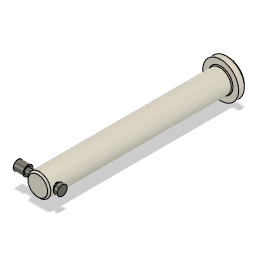
0.885.2200 - Axe pied de hauban - IGTE 21482_225065 (Autodesk Fusion 360 design; units mm, degrees)
Autodesk Fusion 360 part; units mm, degrees
sketch "Sketch1" plane through (0, 0, 0) normal (0, 0, 1) x (1, 0, 0)
  circle A0 centre (0, 0) radius 11
  dimension "d1" = 22
  constraint coincident A0.centre origin
  measures "d1" diameter of A0
extrude "Extrude1" add sketch "Sketch1" along normal blind 4.5 makes body 1
chamfer "Chamfer1" distance 1 angle 45 1 edges at (-10.2556, -3.9778, 0) on bodies 1
sketch "Sketch2" plane through (0, 0, 4.5) normal (0, 0, 1) x (1, 0, 0)
  circle A0 centre (0, 0) radius 11
  circle A1 centre (0, 0) radius 7
  dimension "d5" = 14
  constraint coincident A0.centre A1.centre
  measures "d5" diameter of A1
extrude "Extrude2" add sketch "Sketch2" along normal blind 112 contours A1 bodies 1
fillet "Fillet1" radius 0.5 1 edges at (-6.5263, 2.5313, 4.5) on bodies 1
sketch "Sketch3" plane through (0, 0, 0) normal (1, 0, 0) x (0, 0, -1)
  line L0 (-116.5, 0) -> (-111.5, 0) construction
  circle A0 centre (-111.5, 0) radius 2.5
  point P0 (-116.5, 0)
  dimension "d9" = 5
  dimension "d10" = 5
  constraint coincident P0 L0.start
  constraint coincident L0.end A0.centre
  measures "d9" distance of P0 L0.end
  measures "d10" diameter of A0
extrude "Extrude3" cut sketch "Sketch3" along normal through all and the other way through all bodies 1
chamfer "Chamfer2" distance 1 angle 45 1 edges at (-6.5263, -2.5313, 116.5) on bodies 1
sketch "Sketch4" plane through (0, 0, 0) normal (1, 0, 0) x (0, 0, -1)
  spline S0 degree 3 poles (-111.5, 2.5) (-111.1829, 2.5) (-110.8469, 2.4361) (-110.2319, 2.1801) (-109.9527, 1.9882) (-109.5119, 1.5474) (-109.3199, 1.2682) (-109.0639, 0.653) (-109, 0.3169) (-109, -0.3169) (-109.0639, -0.653) (-109.3199, -1.2682) (-109.5119, -1.5474) (-109.9527, -1.9882) (-110.2319, -2.1801) (-110.8469, -2.4361) (-111.1829, -2.5) (-111.8171, -2.5) (-112.1531, -2.4361) (-112.7681, -2.1801) (-113.0473, -1.9882) (-113.4881, -1.5474) (-113.6801, -1.2682) (-113.9361, -0.653) (-114, -0.3169) (-114, 0.3169) (-113.9361, 0.653) (-113.6801, 1.2682) (-113.4881, 1.5474) (-113.0473, 1.9882) (-112.7681, 2.1801) (-112.1531, 2.4361) (-111.8171, 2.5) (-111.5, 2.5) knots 0 0 0 0 0.095117 0.095117 0.190234 0.190234 0.285292 0.285292 0.38035 0.38035 0.475408 0.475408 0.570466 0.570466 0.665583 0.665583 0.7607 0.7607 0.855818 0.855818 0.950935 0.950935 1.045993 1.045993 1.141051 1.141051 1.236109 1.236109 1.331167 1.331167 1.426284 1.426284 1.521401 1.521401 1.521401 1.521401
  spline S1 degree 3 poles (-111.5, 2.2) (-111.2233, 2.2) (-110.9233, 2.1429) (-110.6547, 2.0311) (-110.3859, 1.9193) (-110.1368, 1.7481) (-109.9444, 1.5556) (-109.752, 1.3633) (-109.5808, 1.1141) (-109.4689, 0.8453) (-109.357, 0.5766) (-109.3, 0.2765) (-109.3, 0) (-109.3, -0.2765) (-109.357, -0.5766) (-109.4689, -0.8453) (-109.5808, -1.1141) (-109.752, -1.3633) (-109.9444, -1.5556) (-110.1368, -1.7481) (-110.3859, -1.9193) (-110.6547, -2.0311) (-110.9233, -2.1429) (-111.2233, -2.2) (-111.5, -2.2) (-111.7767, -2.2) (-112.0767, -2.1429) (-112.3453, -2.0311) (-112.6141, -1.9193) (-112.8632, -1.7481) (-113.0556, -1.5556) (-113.248, -1.3633) (-113.4192, -1.1141) (-113.5311, -0.8453) (-113.643, -0.5766) (-113.7, -0.2765) (-113.7, 0) (-113.7, 0.2765) (-113.643, 0.5766) (-113.5311, 0.8453) (-113.4192, 1.1141) (-113.248, 1.3633) (-113.0556, 1.5556) (-112.8632, 1.7481) (-112.6141, 1.9193) (-112.3453, 2.0311) (-112.0767, 2.1429) (-111.7767, 2.2) (-111.5, 2.2) knots 0 0 0 0 0.095117 0.095117 0.095117 0.190234 0.190234 0.190234 0.285292 0.285292 0.285292 0.38035 0.38035 0.38035 0.475408 0.475408 0.475408 0.570466 0.570466 0.570466 0.665583 0.665583 0.665583 0.7607 0.7607 0.7607 0.855818 0.855818 0.855818 0.950935 0.950935 0.950935 1.045993 1.045993 1.045993 1.141051 1.141051 1.141051 1.236109 1.236109 1.236109 1.331167 1.331167 1.331167 1.426284 1.426284 1.426284 1.521401 1.521401 1.521401 1.521401
  dimension "d14" = 0.3
  measures "d14" distance of S0
extrude "Extrude4" add sketch "Sketch4" along normal blind 10 and the other way blind 17 separate body contours S1 makes body 2
sketch "Sketch5" plane through (10, 0, 0) normal (1, 0, 0) x (0, 0, -1)
  spline S0 degree 3 poles (-111.5, 2.2) (-111.7767, 2.2) (-112.0767, 2.1429) (-112.3453, 2.0311) (-112.6141, 1.9193) (-112.8632, 1.7481) (-113.0556, 1.5556) (-113.248, 1.3633) (-113.4192, 1.1141) (-113.5311, 0.8453) (-113.643, 0.5766) (-113.7, 0.2765) (-113.7, 0) (-113.7, -0.2765) (-113.643, -0.5766) (-113.5311, -0.8453) (-113.4192, -1.1141) (-113.248, -1.3633) (-113.0556, -1.5556) (-112.8632, -1.7481) (-112.6141, -1.9193) (-112.3453, -2.0311) (-112.0767, -2.1429) (-111.7767, -2.2) (-111.5, -2.2) (-111.2233, -2.2) (-110.9233, -2.1429) (-110.6547, -2.0311) (-110.3859, -1.9193) (-110.1368, -1.7481) (-109.9444, -1.5556) (-109.752, -1.3633) (-109.5808, -1.1141) (-109.4689, -0.8453) (-109.357, -0.5766) (-109.3, -0.2765) (-109.3, 0) (-109.3, 0.2765) (-109.357, 0.5766) (-109.4689, 0.8453) (-109.5808, 1.1141) (-109.752, 1.3633) (-109.9444, 1.5556) (-110.1368, 1.7481) (-110.3859, 1.9193) (-110.6547, 2.0311) (-110.9233, 2.1429) (-111.2233, 2.2) (-111.5, 2.2) knots -1.521401 -1.521401 -1.521401 -1.521401 -1.426284 -1.426284 -1.426284 -1.331167 -1.331167 -1.331167 -1.236109 -1.236109 -1.236109 -1.141051 -1.141051 -1.141051 -1.045993 -1.045993 -1.045993 -0.950935 -0.950935 -0.950935 -0.855818 -0.855818 -0.855818 -0.7607 -0.7607 -0.7607 -0.665583 -0.665583 -0.665583 -0.570466 -0.570466 -0.570466 -0.475408 -0.475408 -0.475408 -0.38035 -0.38035 -0.38035 -0.285292 -0.285292 -0.285292 -0.190234 -0.190234 -0.190234 -0.095117 -0.095117 -0.095117 0 0 0 0
  spline S1 degree 3 poles (-111.5, 2.2) (-111.7767, 2.2) (-112.0767, 2.1429) (-112.3453, 2.0311) (-112.6141, 1.9193) (-112.8632, 1.7481) (-113.0556, 1.5556) (-113.248, 1.3633) (-113.4192, 1.1141) (-113.5311, 0.8453) (-113.643, 0.5766) (-113.7, 0.2765) (-113.7, 0) (-113.7, -0.2765) (-113.643, -0.5766) (-113.5311, -0.8453) (-113.4192, -1.1141) (-113.248, -1.3633) (-113.0556, -1.5556) (-112.8632, -1.7481) (-112.6141, -1.9193) (-112.3453, -2.0311) (-112.0767, -2.1429) (-111.7767, -2.2) (-111.5, -2.2) (-111.2233, -2.2) (-110.9233, -2.1429) (-110.6547, -2.0311) (-110.3859, -1.9193) (-110.1368, -1.7481) (-109.9444, -1.5556) (-109.752, -1.3633) (-109.5808, -1.1141) (-109.4689, -0.8453) (-109.357, -0.5766) (-109.3, -0.2765) (-109.3, 0) (-109.3, 0.2765) (-109.357, 0.5766) (-109.4689, 0.8453) (-109.5808, 1.1141) (-109.752, 1.3633) (-109.9444, 1.5556) (-110.1368, 1.7481) (-110.3859, 1.9193) (-110.6547, 2.0311) (-110.9233, 2.1429) (-111.2233, 2.2) (-111.5, 2.2) knots -1.521401 -1.521401 -1.521401 -1.521401 -1.426284 -1.426284 -1.426284 -1.331167 -1.331167 -1.331167 -1.236109 -1.236109 -1.236109 -1.141051 -1.141051 -1.141051 -1.045993 -1.045993 -1.045993 -0.950935 -0.950935 -0.950935 -0.855818 -0.855818 -0.855818 -0.7607 -0.7607 -0.7607 -0.665583 -0.665583 -0.665583 -0.570466 -0.570466 -0.570466 -0.475408 -0.475408 -0.475408 -0.38035 -0.38035 -0.38035 -0.285292 -0.285292 -0.285292 -0.190234 -0.190234 -0.190234 -0.095117 -0.095117 -0.095117 0 0 0 0
  spline S2 degree 3 poles (-111.5, 2.2) (-111.2233, 2.2) (-110.9233, 2.1429) (-110.6547, 2.0311) (-110.3859, 1.9193) (-110.1368, 1.7481) (-109.9444, 1.5556) (-109.752, 1.3633) (-109.5808, 1.1141) (-109.4689, 0.8453) (-109.357, 0.5766) (-109.3, 0.2765) (-109.3, 0) (-109.3, -0.2765) (-109.357, -0.5766) (-109.4689, -0.8453) (-109.5808, -1.1141) (-109.752, -1.3633) (-109.9444, -1.5556) (-110.1368, -1.7481) (-110.3859, -1.9193) (-110.6547, -2.0311) (-110.9233, -2.1429) (-111.2233, -2.2) (-111.5, -2.2) (-111.7767, -2.2) (-112.0767, -2.1429) (-112.3453, -2.0311) (-112.6141, -1.9193) (-112.8632, -1.7481) (-113.0556, -1.5556) (-113.248, -1.3633) (-113.4192, -1.1141) (-113.5311, -0.8453) (-113.643, -0.5766) (-113.7, -0.2765) (-113.7, 0) (-113.7, 0.2765) (-113.643, 0.5766) (-113.5311, 0.8453) (-113.4192, 1.1141) (-113.248, 1.3633) (-113.0556, 1.5556) (-112.8632, 1.7481) (-112.6141, 1.9193) (-112.3453, 2.0311) (-112.0767, 2.1429) (-111.7767, 2.2) (-111.5, 2.2) knots 0 0 0 0 0.095117 0.095117 0.095117 0.190234 0.190234 0.190234 0.285292 0.285292 0.285292 0.38035 0.38035 0.38035 0.475408 0.475408 0.475408 0.570466 0.570466 0.570466 0.665583 0.665583 0.665583 0.7607 0.7607 0.7607 0.855818 0.855818 0.855818 0.950935 0.950935 0.950935 1.045993 1.045993 1.045993 1.141051 1.141051 1.141051 1.236109 1.236109 1.236109 1.331167 1.331167 1.331167 1.426284 1.426284 1.426284 1.521401 1.521401 1.521401 1.521401
  circle A0 centre (-111.5, 0) radius 3
  point P0 (-111.5, 2.2)
  dimension "d19" = 6
  measures "d19" diameter of A0
extrude "Extrude5" add sketch "Sketch5" against normal blind 2.3 contours S0 S1 S2 | A0 bodies 2
sketch "Sketch6" plane through (-17, 0, 0) normal (-1, 0, 0) x (0, 0, 1)
  spline S0 degree 3 poles (111.5, 2.2) (111.2233, 2.2) (110.9233, 2.1429) (110.6547, 2.0311) (110.3859, 1.9193) (110.1368, 1.7481) (109.9444, 1.5556) (109.752, 1.3633) (109.5808, 1.1141) (109.4689, 0.8453) (109.357, 0.5766) (109.3, 0.2765) (109.3, 0) (109.3, -0.2765) (109.357, -0.5766) (109.4689, -0.8453) (109.5808, -1.1141) (109.752, -1.3633) (109.9444, -1.5556) (110.1368, -1.7481) (110.3859, -1.9193) (110.6547, -2.0311) (110.9233, -2.1429) (111.2233, -2.2) (111.5, -2.2) (111.7767, -2.2) (112.0767, -2.1429) (112.3453, -2.0311) (112.6141, -1.9193) (112.8632, -1.7481) (113.0556, -1.5556) (113.248, -1.3633) (113.4192, -1.1141) (113.5311, -0.8453) (113.643, -0.5766) (113.7, -0.2765) (113.7, 0) (113.7, 0.2765) (113.643, 0.5766) (113.5311, 0.8453) (113.4192, 1.1141) (113.248, 1.3633) (113.0556, 1.5556) (112.8632, 1.7481) (112.6141, 1.9193) (112.3453, 2.0311) (112.0767, 2.1429) (111.7767, 2.2) (111.5, 2.2) knots 0 0 0 0 0.095117 0.095117 0.095117 0.190234 0.190234 0.190234 0.285292 0.285292 0.285292 0.38035 0.38035 0.38035 0.475408 0.475408 0.475408 0.570466 0.570466 0.570466 0.665583 0.665583 0.665583 0.7607 0.7607 0.7607 0.855818 0.855818 0.855818 0.950935 0.950935 0.950935 1.045993 1.045993 1.045993 1.141051 1.141051 1.141051 1.236109 1.236109 1.236109 1.331167 1.331167 1.331167 1.426284 1.426284 1.426284 1.521401 1.521401 1.521401 1.521401
  spline S1 degree 3 poles (111.5, 2.2) (111.4677, 2.1998) (111.4353, 2.1992) (111.1486, 2.1858) (110.8625, 2.122) (110.3144, 1.8831) (110.0981, 1.7094) (109.9444, 1.5556) (109.8214, 1.4326) (109.7114, 1.2909) (109.4765, 0.9058) (109.43, 0.7525) (109.3181, 0.3857) (109.2816, 0.0841) (109.3377, -0.4851) (109.4212, -0.7753) (109.6832, -1.2685) (109.8714, -1.5088) (110.3142, -1.8722) (110.5754, -2.0164) (111.1039, -2.1798) (111.4061, -2.2181) (111.9714, -2.1648) (112.2628, -2.0835) (112.7542, -1.8261) (112.9972, -1.6395) (113.3592, -1.2045) (113.5073, -0.9446) (113.6735, -0.4247) (113.717, -0.1208) (113.671, 0.4363) (113.5949, 0.7304) (113.3527, 1.212) (113.1703, 1.4637) (112.7547, 1.8231) (112.4982, 1.981) (112.0701, 2.1313) (111.7856, 2.1974) (111.5, 2.2) knots -0.122125 -0.122125 -0.122125 -0.122125 -0.115736 -0.115736 -0.065218 -0.065218 0 0 0 0.052189 0.052189 0.134842 0.134842 0.34423 0.34423 0.542353 0.542353 0.733658 0.733658 0.91385 0.91385 1.08848 1.08848 1.25086 1.25086 1.405126 1.405126 1.546294 1.546294 1.679136 1.679136 1.797637 1.797637 1.905712 1.905712 1.996221 1.996221 2.052666 2.052666 2.052666 2.052666 construction
  spline S2 degree 3 poles (111.5, 2.2) (111.2233, 2.2) (110.9233, 2.1429) (110.6547, 2.0311) (110.3859, 1.9193) (110.1368, 1.7481) (109.9444, 1.5556) (109.752, 1.3633) (109.5808, 1.1141) (109.4689, 0.8453) (109.357, 0.5766) (109.3, 0.2765) (109.3, 0) (109.3, -0.2765) (109.357, -0.5766) (109.4689, -0.8453) (109.5808, -1.1141) (109.752, -1.3633) (109.9444, -1.5556) (110.1368, -1.7481) (110.3859, -1.9193) (110.6547, -2.0311) (110.9233, -2.1429) (111.2233, -2.2) (111.5, -2.2) (111.7767, -2.2) (112.0767, -2.1429) (112.3453, -2.0311) (112.6141, -1.9193) (112.8632, -1.7481) (113.0556, -1.5556) (113.248, -1.3633) (113.4192, -1.1141) (113.5311, -0.8453) (113.643, -0.5766) (113.7, -0.2765) (113.7, 0) (113.7, 0.2765) (113.643, 0.5766) (113.5311, 0.8453) (113.4192, 1.1141) (113.248, 1.3633) (113.0556, 1.5556) (112.8632, 1.7481) (112.6141, 1.9193) (112.3453, 2.0311) (112.0767, 2.1429) (111.7767, 2.2) (111.5, 2.2) knots 0 0 0 0 0.095117 0.095117 0.095117 0.190234 0.190234 0.190234 0.285292 0.285292 0.285292 0.38035 0.38035 0.38035 0.475408 0.475408 0.475408 0.570466 0.570466 0.570466 0.665583 0.665583 0.665583 0.7607 0.7607 0.7607 0.855818 0.855818 0.855818 0.950935 0.950935 0.950935 1.045993 1.045993 1.045993 1.141051 1.141051 1.141051 1.236109 1.236109 1.236109 1.331167 1.331167 1.331167 1.426284 1.426284 1.426284 1.521401 1.521401 1.521401 1.521401
  circle A0 centre (111.5, 0) radius 3
  point P0 (111.5, 2.2)
  dimension "d22" = 6
  measures "d22" diameter of A0
extrude "Extrude6" add sketch "Sketch6" against normal blind 6 bodies 2
